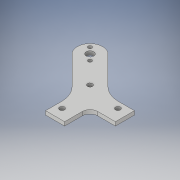
# Autodesk Inventor part: quarter_upper
Saved by Autodesk Inventor 2019 (Build 230136000, 136)
## iProperties
Created: 2019-01-09
Part Number: quarter_upper
Material: Generic
Document SubType Name: Modeling
Designer: Daniel
Density: 1 g/cm^3
Appearance: Default
Author: Daniel
Autodesk Inventor part; units mm, degrees
ref_plane "YZ Plane" through (0, 0, 0) normal (1, 0, 0) x (0, 1, 0)
ref_plane "XZ Plane" through (0, 0, 0) normal (0, 1, 0) x (-1, 0, 0)
ref_plane "XY Plane" through (0, 0, 0) normal (0, 0, 1) x (1, 0, 0)
sketch "Sketch23" plane through (0, 0, 0) normal (0, 1, 0) x (-1, 0, 0)
  line L0 (0, -7) -> (0, 42) projected
  line L1 (7, 0) -> (-42, 0) projected
  line L2 (0, 0) -> (-35, 0)
  line L3 (-35, 0) -> (-35, 35)
  line L4 (-35, 35) -> (0, 35)
  line L5 (0, 35) -> (0, 0)
  line L6 (0, 0) -> (-35, 35) construction
  point P0 (0, 0)
  dimension "d213" = 35
  dimension "d214" = 35
  constraints: 10 end point, 2 collinear, 2 parallel, 1 horizontal, 1 perpendicular
  measures "d213" distance between parallel lines of L3 L5
  measures "d214" distance between parallel lines of L4 L2
extrude "Extrusion14" add sketch "Sketch23" along normal blind 3
sketch "Sketch24" plane through (0, 3, 0) normal (0, 1, 0) x (1, 0, 0)
  line L0 (35, 0) -> (0, 0) projected
  line L1 (0, 0) -> (0, -35) projected
  line L2 (0, -35) -> (35, -35) projected
  line L3 (35, -35) -> (35, 0) projected
  line L4 (-41.7276, 41.7276) -> (35, -35) construction
  line L5 (-35.3553, 21.2132) -> (-21.2132, 35.3553)
  line L6 (-21.2132, 35.3553) -> (14.1421, 0)
  line L7 (35, 0) -> (0, 0) projected
  line L8 (0, -14.1421) -> (-35.3553, 21.2132)
  line L9 (-23.915, -23.915) -> (42.6519, 42.6519) construction
  dimension "d217" = 45
  dimension "d218" = 20
  dimension "d219" = 40
  constraints: 10 end point, 4 point on line, 3 parallel, 1 other
  measures "d217" angle of L0 L9
  measures "d218" distance between parallel lines of L8 L6
  measures "d219" distance between parallel lines of L9 L5
extrude "Extrusion15" add sketch "Sketch24" against normal blind 3 contours L0 L1 L8 L5 L6
sketch "Sketch36" plane through (0, 3, 0) normal (0, 1, 0) x (1, 0, 0)
  line L0 (-35.3553, 21.2132) -> (0, -14.1421) projected
  line L1 (14.1421, 0) -> (-21.2132, 35.3553) projected
  line L2 (-21.2132, 35.3553) -> (-35.3553, 21.2132) projected
  line L3 (-24.0416, 32.5269) -> (-32.5269, 24.0416) projected
  line L4 (20, -20) -> (32, -20) projected
  line L5 (-18.4468, 18.4468) -> (20, -20) construction
  line L6 (-49.4264, 0) -> (49.0711, 0) projected
  line L7 (0, 49.4264) -> (0, -49.0711) projected
  line L8 (35, 0) -> (14.1421, 0) projected
  line L9 (0, -14.1421) -> (0, -35) projected
  line L10 (35, -35) -> (35, 0) projected
  line L11 (0, -35) -> (35, -35) projected
  point P0 (0, 0)
  point P1 (-18.3848, 9.8995)
  point P2 (0, -32)
  point P3 (32, 0)
  point P4 (-9.8995, 18.3848)
  point P5 (-21.2132, 21.2132)
  dimension "d311" = 45
  dimension "d312" = 10
  constraints: 2 end point, 1 point on line
  measures "d311" angle of L6 L5
  measures "d312" distance from line of L3 point (-21.213, 21.213)
hole "Hole17" at (-21.2132, 3, -21.2132) direction (0, -1, 0) diameter 6 end through all
sketch "Sketch37" plane through (0, 3, 0) normal (0, 1, 0) x (1, 0, 0)
  circle A0 centre (-21.2132, 21.2132) radius 3 projected
  line L0 (14.1421, 0) -> (-21.2132, 35.3553) projected
  line L1 (-21.2132, 35.3553) -> (-35.3553, 21.2132) projected
  line L2 (-35.3553, 21.2132) -> (0, -14.1421) projected
  line L3 (-34.5369, 34.5369) -> (-7.0609, 7.0609) construction
  line L4 (-38.7653, 3.6611) -> (1.6595, 44.0859) construction
  line L5 (-53.5184, 0) -> (49.7531, 0) projected
  line L6 (0, 59.903) -> (0, -50.8172) projected
  line L7 (35, 0) -> (14.1421, 0) projected
  line L8 (0, -14.1421) -> (0, -35) projected
  line L9 (35, -35) -> (35, 0) projected
  line L10 (0, -35) -> (35, -35) projected
  point P0 (0, 0)
  point P1 (32, 0)
  point P2 (0, -32)
  point P3 (-25.8094, 25.8094)
  point P4 (-16.617, 16.617)
  dimension "d321" = 45
  dimension "d322" = 45
  dimension "d323" = 6.5
  dimension "d324" = 6.5
  constraints: 4 end point, 4 point on line
  measures "d321" angle of L5 L4
  measures "d322" angle of L5 L3
  measures "d323" distance from line of L4 point (-25.809, 25.809)
  measures "d324" distance from line of L4 point (-16.617, 16.617)
hole "Hole18" at (-25.8094, 3, -25.8094) at (-16.617, 3, -16.617) direction (0, -1, 0) diameter 3 end through all
fillet "Fillet15" radius 10 2 edges at (-35.3553, 1.5, -21.2132) (-21.2132, 1.5, -35.3553)
fillet "Fillet18" radius 20 2 edges at (14.1421, 1.5, 0) (0, 1.5, 14.1421)
sketch "Sketch39" plane through (0, 3, 0) normal (0, 1, 0) x (1, 0, 0)
  circle A0 centre (-21.2132, 21.2132) radius 3 projected
  circle A1 centre (-16.617, 16.617) radius 1.5 projected
  circle A2 centre (-25.8094, 25.8094) radius 1.5 projected
  arc A3 (-14.1421, 28.2843) -> (-28.2843, 14.1421) centre (-21.2132, 21.2132) ccw projected
  line L0 (-28.2843, 14.1421) -> (-5.8579, -8.2843) projected
  arc A4 (0, -22.4264) -> (-5.8579, -8.2843) centre (-20, -22.4264) ccw projected
  line L1 (0, -22.4264) -> (0, -35) projected
  line L2 (35, 0) -> (22.4264, 0) projected
  arc A5 (8.2843, 5.8579) -> (22.4264, 0) centre (22.4264, 20) ccw projected
  line L3 (8.2843, 5.8579) -> (-14.1421, 28.2843) projected
  line L4 (26.8786, -26.8786) -> (-35.1686, 35.1686) construction
  line L5 (-58.6564, 0) -> (50.6094, 0) projected
  line L6 (0, 49.4264) -> (0, -49.0711) projected
  line L7 (-9.3628, 33.0636) -> (-43.047, -0.6206) construction
  line L8 (0, -35) -> (35, -35) projected
  line L9 (35, -35) -> (35, 0) projected
  point P0 (0, 0)
  point P1 (0, -32)
  point P2 (32, 0)
  point P3 (0, 0)
  dimension "d339" = 45
  dimension "d340" = 30
  constraints: 4 end point, 3 point on line, 1 perpendicular
  measures "d339" angle of L5 L4
  measures "d340" distance from line of L7 point (0, 0)
hole "Hole19" at (0, 3, 0) direction (0, -1, 0) diameter 4 end through all
sketch "Sketch40" plane through (0, 3, 0) normal (0, 1, 0) x (1, 0, 0)
  circle A0 centre (0, 0) radius 2 projected
  circle A1 centre (-25.8094, 25.8094) radius 1.5 projected
  circle A2 centre (-16.617, 16.617) radius 1.5 projected
  circle A3 centre (-21.2132, 21.2132) radius 3 projected
  arc A4 (-14.1421, 28.2843) -> (-28.2843, 14.1421) centre (-21.2132, 21.2132) ccw projected
  line L0 (-28.2843, 14.1421) -> (-5.8579, -8.2843) projected
  arc A5 (0, -22.4264) -> (-5.8579, -8.2843) centre (-20, -22.4264) ccw projected
  line L1 (0, -22.4264) -> (0, -35) projected
  line L2 (0, -35) -> (35, -35) projected
  line L3 (35, -35) -> (35, 0) projected
  line L4 (35, 0) -> (22.4264, 0) projected
  arc A6 (8.2843, 5.8579) -> (22.4264, 0) centre (22.4264, 20) ccw projected
  line L5 (8.2843, 5.8579) -> (-14.1421, 28.2843) projected
  line L6 (35, -35) -> (15, -35)
  line L7 (15, -35) -> (15, -15)
  line L8 (15, -15) -> (35, -15)
  line L9 (35, -15) -> (35, -35)
  line L10 (0, -35) -> (35, -35) projected
  line L11 (35, -35) -> (35, 0) projected
  point P0 (0, 0)
  dimension "d394" = 15
  dimension "d395" = 15
  constraints: 8 end point, 2 collinear, 2 parallel, 1 horizontal, 1 perpendicular
  measures "d394" distance between parallel lines of L1 L7
  measures "d395" distance between parallel lines of L4 L8
extrude "Extrusion19" cut sketch "Sketch40" against normal blind 10 contours L3 L2 L7 L8
fillet "Fillet19" radius 6 1 edges at (15, 1.5, 15)
sketch "Sketch44" plane through (0, 3, 0) normal (0, 1, 0) x (1, 0, 0)
  line L0 (15, -35) -> (15, -21) projected
  arc A0 (21, -15) -> (15, -21) centre (21, -21) ccw projected
  line L1 (21, -15) -> (35, -15) projected
  line L2 (35, 0) -> (22.4264, 0) projected
  arc A1 (8.2843, 5.8579) -> (22.4264, 0) centre (22.4264, 20) ccw projected
  line L3 (8.2843, 5.8579) -> (-14.1421, 28.2843) projected
  arc A2 (-14.1421, 28.2843) -> (-28.2843, 14.1421) centre (-21.2132, 21.2132) ccw projected
  line L4 (-28.2843, 14.1421) -> (-5.8579, -8.2843) projected
  arc A3 (0, -22.4264) -> (-5.8579, -8.2843) centre (-20, -22.4264) ccw projected
  line L5 (0, -22.4264) -> (0, -35) projected
  circle A4 centre (-21.2132, 21.2132) radius 3 projected
  circle A5 centre (-16.617, 16.617) radius 1.5 projected
  circle A6 centre (-25.8094, 25.8094) radius 1.5 projected
  circle A7 centre (0, 0) radius 2 projected
  line L6 (35, -15) -> (35, 0) projected
  line L7 (0, -35) -> (15, -35) projected
  point P0 (0, 0)
  point P1 (27, -5)
  point P2 (5, -27)
  dimension "d383" = 5
  dimension "d385" = 5
  measures "d383" distance from line of L2 point (27, -5)
  measures "d385" distance from line of L5 point (5, -27)
hole "Hole22" at (27, 3, 5) at (5, 3, 27) direction (0, -1, 0) diameter 4 end through all
body "Solid5"
